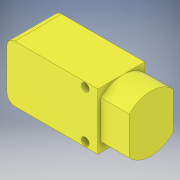
# Autodesk Inventor part: MotorFrame
Saved by Autodesk Inventor 2018 (Build 220112000, 112)
## iProperties
Created: 2018-01-12
Part Number: MotorFrame
Material: ABS Plastic
Document SubType Name: Modeling
Designer: Kyle
Density: 1.06 g/cm^3
Appearance: Smooth - Yellow
Author: Kyle
Autodesk Inventor part; units mm, degrees
ref_plane "YZ Plane" through (0, 0, 0) normal (1, 0, 0) x (0, 1, 0)
ref_plane "XZ Plane" through (0, 0, 0) normal (0, 1, 0) x (-1, 0, 0)
ref_plane "XY Plane" through (0, 0, 0) normal (0, 0, 1) x (1, 0, 0)
sketch "Sketch1" plane through (0, 0, 0) normal (0, 0, 1) x (1, 0, 0)
  line L0 (0, 0) -> (36.83, 0)
  line L1 (36.83, 0) -> (36.83, -22.86)
  line L2 (36.83, -22.86) -> (0, -22.86)
  line L3 (0, -22.86) -> (0, 0)
  dimension "d0" = 36.83
  dimension "d1" = 22.86
  constraints: 8 end point, 2 parallel, 1 horizontal, 1 perpendicular
  measures "d0" distance of L0.start L0.end
  measures "d1" distance of L2.end L0.start
extrude "Extrusion1" add sketch "Sketch1" along normal blind 19.05
fillet "Fillet1" radius 3.175 2 edges at (0, 0, 9.525) (0, -22.86, 9.525)
sketch "Sketch2" plane through (36.83, -22.86, 0) normal (1, 0, 0) x (0, 0, -1)
  line L0 (0, 22.86) -> (-19.05, 22.86) projected
  line L1 (0, 0) -> (-19.05, 0) projected
  line L2 (-19.05, 0) -> (-19.05, 22.86) projected
  arc A0 (0, 19.05) -> (-17.78, 19.1328) centre (-8.93, 10.4897) ccw
  arc A1 (-17.78, 3.81) -> (0, 3.81) centre (-8.89, 12.2767) ccw
  line L3 (0, 19.05) -> (0, 3.81)
  line L4 (0, 22.86) -> (0, 0) projected
  line L5 (-19.05, 3.175) -> (0, 3.175) projected
  line L6 (-17.78, 3.81) -> (-17.78, 19.1328)
  dimension "d5" = 3.81
  dimension "d6" = 3.81
  dimension "d7" = 1.27
  dimension "d8" = 1.27
  constraints: 4 end point, 4 point on circle, 2 centre point, 2 tangent, 1 collinear
  measures "d5" distance from line of L3.start L0
  measures "d6" distance from line of L1 L3.end
  measures "d7" distance from line of L2 L6.start
  measures "d8" distance from line of L2 L6.end
extrude "Extrusion2" add sketch "Sketch2" along normal blind 11.43 contours A0 L3 A1 L5 L6 | A1 L5
sketch "Sketch3" plane through (0, 0, 19.05) normal (0, 0, 1) x (1, 0, 0)
  circle A0 centre (31.75, -1.905) radius 1.5875
  line L0 (36.83, -22.86) -> (36.83, 0) projected
  line L1 (36.83, 0) -> (3.175, 0) projected
  circle A1 centre (31.75, -20.955) radius 1.5875
  line L2 (3.175, -22.86) -> (36.83, -22.86) projected
  point P0 (0, 0)
  dimension "d11" = 3.175
  dimension "d12" = 5.08
  dimension "d13" = 1.905
  dimension "d14" = 1.905
  dimension "d15" = 3.175
  constraints: 2 centre point
  measures "d11" diameter of A0
  measures "d12" distance from line of A0.centre L0
  measures "d13" distance from line of L1 A0.centre
  measures "d14" distance from line of L2 A1.centre
  measures "d15" diameter of A1
extrude "Extrusion3" cut sketch "Sketch3" against normal blind 25.4
body "Solid1"
